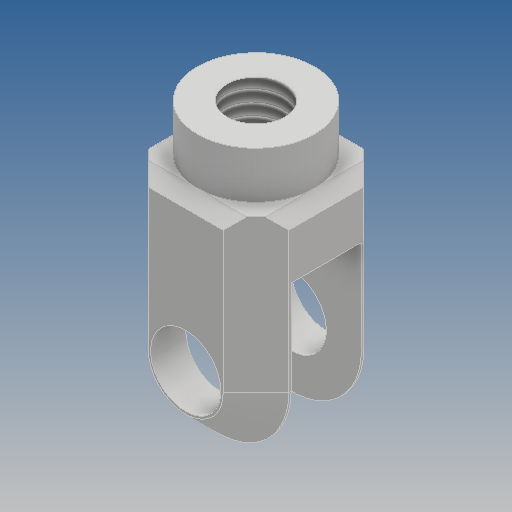
# Autodesk Inventor part: Gabel
Saved by Autodesk Inventor 2018 (Build 220112000, 112)
## iProperties
Created: 2018-10-23
Part Number: Gabel
Material: Generisch
Document SubType Name: Modeling
Designer: M.Knabel
Density: 1 g/cm^3
Appearance: Vorgabe
Mass: 0.158259 g
Surface Area: 3.27503 cm^2
Volume: 0.158259 cm^3
Author: M.Knabel
Autodesk Inventor part; units mm, degrees
ref_plane "YZ Plane" through (0, 0, 0) normal (1, 0, 0) x (0, 1, 0)
ref_plane "XZ Plane" through (0, 0, 0) normal (0, 1, 0) x (-1, 0, 0)
ref_plane "XY Plane" through (0, 0, 0) normal (0, 0, 1) x (1, 0, 0)
sketch "Skizze1" plane through (0, 0, 0) normal (0, 0, 1) x (1, 0, 0)
  line L0 (0, -1.2) -> (0, 7.2) projected
  line L1 (-1.2, 0) -> (7.2, 0) projected
  line L2 (0, 0) -> (6, 0)
  line L3 (6, 0) -> (6, 6)
  line L4 (6, 6) -> (0, 6)
  line L5 (0, 6) -> (0, 0)
  dimension "d0" = 6
  dimension "d1" = 6
  constraints: 8 end point, 2 parallel, 1 horizontal, 1 perpendicular
  measures "d0" distance between parallel lines of L3 L0
  measures "d1" distance between parallel lines of L1 L4
extrude "Extrusion1" add sketch "Skizze1" along normal blind 9.5
sketch "Skizze2" plane through (0, 0, 9.5) normal (0, 0, 1) x (1, 0, 0)
  line L0 (0, 0) -> (6, 0) projected
  line L1 (6, 0) -> (6, 6) projected
  line L2 (6, 6) -> (0, 6) projected
  line L3 (0, 6) -> (0, 0) projected
  circle A0 centre (3, 3) radius 2.5
  dimension "d4" = 5
  dimension "d5" = 3
  dimension "d6" = 3
  constraints: 1 centre point
  measures "d4" diameter of A0
  measures "d5" distance from line of L3 A0.centre
  measures "d6" distance from line of A0.centre L2
extrude "Extrusion2" add sketch "Skizze2" along normal blind 2 contours A0
sketch "Skizze3" plane through (0, 0, 0) normal (-1, 0, 0) x (0, 0, 1)
  line L0 (0, -1.2) -> (0, 7.2) projected
  line L1 (-2.3, 0) -> (13.8, 0) projected
  line L2 (0, 0) -> (0, 6) projected
  line L3 (0, 4.5) -> (7, 4.5)
  line L4 (7, 4.5) -> (7, 1.5)
  line L5 (7, 1.5) -> (0, 1.5)
  line L6 (0, 1.5) -> (0, 4.5)
  dimension "d12" = 1.5
  dimension "d13" = 3
  dimension "d14" = 7
  constraints: 8 end point, 2 parallel, 1 horizontal, 1 perpendicular, 1 point on line
  measures "d12" distance between parallel lines of L1 L5
  measures "d13" distance between parallel lines of L5 L3
  measures "d14" distance between parallel lines of L0 L4
extrude "Extrusion3" cut sketch "Skizze3" against normal through all
chamfer "Fase2" distance 0.5 angle 45 4 edges at (6, 3, 9.5) (3, 0, 9.5) (3, 6, 9.5) (0, 3, 9.5)
sketch "Skizze4" plane through (0, 0, 0) normal (0, -1, 0) x (1, 0, 0)
  line L0 (0, 9) -> (6, 9) projected
  line L1 (0, 0) -> (0, 9) projected
  line L2 (0, 0) -> (6, 0) projected
  line L3 (6, 0) -> (6, 9) projected
  point P0 (3, 3)
  dimension "d20" = 3
  dimension "d21" = 3
  measures "d20" distance from line of L2 point (3, 3)
  measures "d21" distance from line of point (3, 3) L1
hole "Bohrung1" at (3, 0, 3) direction (0, 1, 0) diameter 3 end up to face face through (4, 6, 6) facing (0, 1, 0)
sketch "Skizze5" plane through (3, 3, 11.5) normal (0, 0, 1) x (1, 0, 0)
  circle A0 centre (0, 0) radius 2.5 projected
  point P0 (-3, -3)
  constraints: 1 coincident
hole "Bohrung2" at (3, 3, 11.5) direction (0, 0, -1) diameter 2.459 end through all thread size "M3x0.5" class "6H" standard "ISO Metric profile"
sketch "Skizze7" plane through (0, 0, 0) normal (0, -1, 0) x (1, 0, 0)
  circle A0 centre (3, 3) radius 1.5 projected
  line L0 (0, 9) -> (6, 9) projected
  line L1 (0, 0) -> (0, 9) projected
  line L2 (0, 0) -> (6, 0) projected
  line L3 (6, 0) -> (6, 9) projected
  arc A1 (0, 3) -> (6, 3) centre (3, 3) ccw
  line L4 (0, 0) -> (0, 7) projected
  line L5 (0, 3) -> (0, -0.5644)
  line L6 (0, -0.5644) -> (6, -0.5644)
  line L7 (6, -0.5644) -> (6, 3)
  line L8 (6, 7) -> (6, 0) projected
  constraints: 6 end point, 2 point on circle, 2 point on line, 1 centre point, 1 coincident, 1 collinear, 1 perpendicular, 1 tangent
extrude "Extrusion4" cut sketch "Skizze7" against normal through all contours A1 L2 L1 | L3 L2 A1 | L2 L7 L6 L5
chamfer "Fase4" distance 1.4 angle 45 6 edges at (3, 0, 0) (6, 0, 6.0001) (0, 0, 6.0001) (3, 6, 0) (0, 6, 6.0001) (6, 6, 6.0001)
